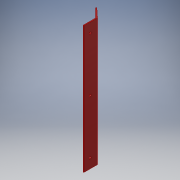
# Autodesk Inventor part: LED strip mount
Saved by Autodesk Inventor 2018 (Build 220112000, 112)
## iProperties
Created: 2017-10-14
Part Number: LED strip mount
Material: ABS-Kunststoff
Document SubType Name: Modeling
Designer: Till
Density: 1.06 g/cm^3
Appearance: Rot
Author: Till
Autodesk Inventor part; units mm, degrees
ref_plane "YZ Plane" through (0, 0, 0) normal (1, 0, 0) x (0, 1, 0)
ref_plane "XZ Plane" through (0, 0, 0) normal (0, 1, 0) x (-1, 0, 0)
ref_plane "XY Plane" through (0, 0, 0) normal (0, 0, 1) x (1, 0, 0)
sketch "Skizze1" plane through (0, 0, 0) normal (0, 0, 1) x (1, 0, 0)
  line L0 (0, -0.8284) -> (0, -20)
  line L1 (0, 0) -> (19.1716, 0) construction
  line L2 (0, -20) -> (1.5, -20)
  line L3 (1.5, -20) -> (1.5, 1.5)
  line L4 (-0.5858, 0.5858) -> (-14.1421, 14.1421)
  line L5 (-14.1421, 14.1421) -> (-13.0815, 15.2028)
  line L6 (-13.0815, 15.2028) -> (1.5, 1.5)
  arc A0 (0, -0.8284) -> (-0.5858, 0.5858) centre (-2, -0.8284) ccw
  dimension "d0" = 20
  dimension "d1" = 90
  dimension "d2" = 1.5
  dimension "d3" = 90
  dimension "d4" = 21.5
  dimension "d5" = 20
  dimension "d6" = 135
  dimension "d7" = 2
  constraints: 14 end point, 4 perpendicular, 3 point on line, 2 point on circle, 2 tangent, 1 centre point, 1 horizontal, 1 vertical
  measures "d0" distance of L1.start L0.end
  measures "d1" angle of L0 L1
  measures "d2" distance of L0.end L2.end
  measures "d3" angle of L2 L0
  measures "d4" distance of L2.end L3.end
  measures "d5" distance of L1.start L4.end
  measures "d6" angle of L4 L0
  measures "d7" radius of A0
extrude "Extrusion1" add sketch "Skizze1" along normal blind 200
hole "Bohrung1" at (1.5, -10, 185) direction (-1, 0, 0) diameter 3.2 end through all
pattern_linear "Rechteckige Anordnung1" count 3 spacing 85 along (0, 0, -1) of "Bohrung1"
fillet "Rundung1" radius 0.69 5 edges at (1.5, -20, 100) (0, -20, 100) (-14.1421, 14.1421, 100) (1.5, 1.5, 100) (-13.0815, 15.2028, 100)
